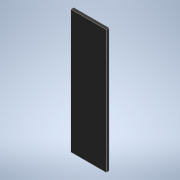
# Autodesk Inventor part: 103.019.01_Daempfer_Stopper
Saved by Autodesk Inventor 2021 (Build 250183000, 183)
## iProperties
Created: 2021-12-02
Part Number: 103.019.01_Daempfer_Stopper
Material: Gummi
Document SubType Name: Modeling
Designer: Sebastian Seewald
Mass: 0.06975 g
Surface Area: 3.31 cm^2
Volume: 0.075 cm^3
Density: 0.93 g/cm^3
Appearance: Gummi - Schwarz
Author: Sebastian Seewald
Autodesk Inventor part; units mm, degrees
ref_plane "YZ Plane" through (0, 0, 0) normal (1, 0, 0) x (0, 1, 0)
ref_plane "XZ Plane" through (0, 0, 0) normal (0, 1, 0) x (-1, 0, 0)
ref_plane "XY Plane" through (0, 0, 0) normal (0, 0, 1) x (1, 0, 0)
sketch "Skizze1" plane through (0, 0, 0) normal (0, 0, 1) x (1, 0, 0)
  line L0 (0, 0) -> (6, 0)
  line L1 (6, 0) -> (6, 21)
  line L2 (6, 21) -> (0, 21)
  line L3 (0, 21) -> (0, 0)
  dimension "d0" = 21
  dimension "d1" = 6
  constraints: 8 end point, 2 parallel, 1 horizontal, 1 perpendicular
  measures "d0" distance between parallel lines of L0 L2
  measures "d1" distance between parallel lines of L3 L1
extrude "Extrusion1" add sketch "Skizze1" along normal blind 0.5
